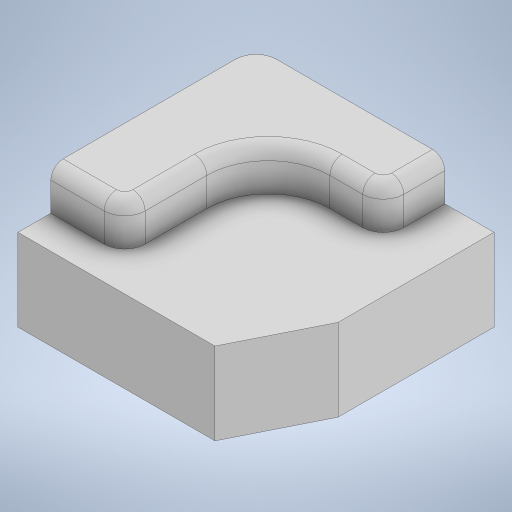
# Autodesk Inventor part: primo esercizio
Saved by Autodesk Inventor 2023 (Build 270158000, 158)
## iProperties
Created: 2023-02-13
Part Number: primo esercizio
Material: Generico
Document SubType Name: Modeling
Designer: Admin
Density: 1 g/cm^3
Appearance: Default
Author: Admin
Autodesk Inventor part; units mm, degrees
ref_plane "YZ Plane" through (0, 0, 0) normal (1, 0, 0) x (0, 1, 0)
ref_plane "XZ Plane" through (0, 0, 0) normal (0, 1, 0) x (-1, 0, 0)
ref_plane "XY Plane" through (0, 0, 0) normal (0, 0, 1) x (1, 0, 0)
sketch "Schizzo11" plane through (0, 0, 0) normal (0, 1, 0) x (-1, 0, 0)
  line L0 (29, -29) -> (-29, -29)
  line L1 (-29, -29) -> (-29, 9)
  line L2 (-19, 29) -> (29, 29)
  line L3 (29, 29) -> (29, -29)
  line L4 (29, -29) -> (-29, 29) construction
  line L5 (-29, -29) -> (29, 29) construction
  line L6 (29, -29) -> (29, 21)
  line L7 (29, 21) -> (16, 21)
  line L8 (11, 16) -> (11, 1)
  line L9 (29, -29) -> (-17, -29)
  line L10 (-17, -29) -> (-17, -19)
  line L11 (-12, -14) -> (-4, -14)
  arc A0 (-4, -14) -> (11, 1) centre (-4, 1) ccw
  arc A1 (16, 21) -> (11, 16) centre (16, 16) ccw
  arc A2 (-12, -14) -> (-17, -19) centre (-12, -19) ccw
  line L12 (-19, 29) -> (-29, 9)
  point P0 (0, 0)
  point P1 (11, 21)
  point P2 (11, -14)
  point P3 (-17, -14)
  dimension "d28" = 58
  dimension "d29" = 58
  dimension "d30" = 50
  dimension "d31" = 18
  dimension "d32" = 35
  dimension "d33" = 46
  dimension "d34" = 15
  dimension "d35" = 15
  dimension "d36" = 5
  dimension "d37" = 5
  dimension "d38" = 10
  dimension "d39" = 20
  constraints: 26 end point, 10 point on line, 6 point on circle, 6 tangent, 4 perpendicular, 3 centre point, 2 midpoint, 2 parallel, 1 horizontal
  measures "d28" distance of L4.end L2.end
  measures "d29" distance of L0.end L4.end
  measures "d30" distance of L0.start L6.end
  measures "d31" distance of L6.end point (11, 21)
  measures "d32" distance of point (11, 21) point (11, -14)
  measures "d33" distance of L0.start L9.end
  measures "d34" distance of L9.end point (-17, -14)
  measures "d35" radius of A0
  measures "d36" radius of A1
  measures "d37" radius of A2
  measures "d38" distance of L2.start L4.end
  measures "d39" distance of L1.end L4.end
extrude "Estrusione6" add sketch "Schizzo11" along normal blind 30 contours L0 L10 A2 L11 A0 L8 A1 L7 L3
extrude "Estrusione7" add sketch "Schizzo11" along normal blind 20 contours L0 L1 L12 L2 L3 L7 A1 L8 A0 L11 A2 L10
fillet "Raccordo3" radius 3 7 edges at (8, 30, -14) (15.5355, 30, -15.4645) (17, 30, -24) (-11, 30, 8.5) (-12.4645, 30, 19.5355) (-22.5, 30, 21) (-6.6066, 30, -9.6066)
fillet "Raccordo4" radius 5 1 edges at (-29, 15, -29)
